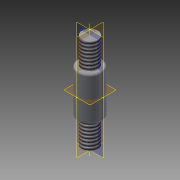
# Autodesk Inventor part: SchleppstangeBefestigung
Saved by Autodesk Inventor 2015 (Build 190159000, 159)
## iProperties
Created: 2018-11-19
Part Number: SchleppstangeBefestigung
Material: Generisch
Document SubType Name: Modeling
Designer: Boris
Density: 1 g/cm^3
Appearance: Vorgabe
Author: Boris
Autodesk Inventor part; units mm, degrees
sketch "Skizze1" plane through (0, 0, 0) normal (0, 0, 1) x (1, 0, 0)
  circle A0 centre (0, 0) radius 1.5
  dimension "d0" = 3
  constraints: 1 centre point, 1 coincident
  measures "d0" diameter of A0
extrude "Extrusion1" add sketch "Skizze1" along normal mid plane 12
sketch "Skizze2" plane through (0, 0, 6) normal (0, 0, 1) x (1, 0, 0)
  circle A0 centre (0, 0) radius 1
  circle A1 centre (0, 0) radius 1.5 projected
  dimension "d3" = 2
  constraints: 1 centre point, 1 coincident
  measures "d3" diameter of A0
extrude "Extrusion2" cut sketch "Skizze2" against normal blind 3.25
thread "Gewinde2" size "M2x0.4" class "6g" standard "ANSI Metric M Profile" full length
mirror "Spiegeln1" about plane through (0, 0, 0) normal (0, 0, 1) of "Extrusion2"
fillet "Rundung1" radius 0.25 2 edges at (-1.5, 0, 2.75) (-1.5, 0, -2.75)
